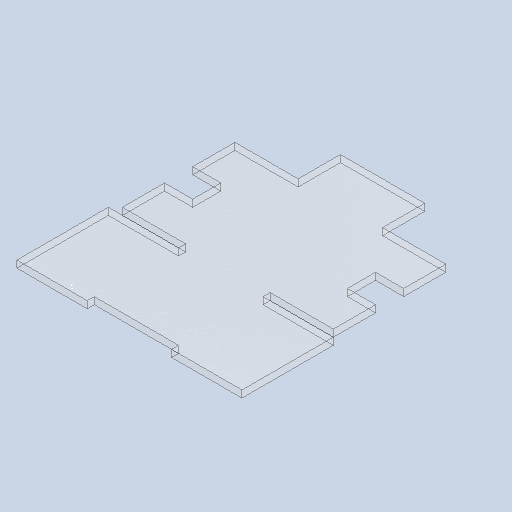
# Autodesk Inventor part: HOOD_1
Saved by Autodesk Inventor 2025.3 (Build 293356030, 356C)
## iProperties
Created: 2026-06-30
Part Number: HOOD_1
Material: Acrylic
Document SubType Name: Modeling
Designer: user
Density: 1.188 g/cm^3
Appearance: Transparent - Clear
Author: user
Autodesk Inventor part; units mm, degrees
ref_plane "YZ Plane" through (0, 0, 0) normal (1, 0, 0) x (0, 1, 0)
ref_plane "XZ Plane" through (0, 0, 0) normal (0, 1, 0) x (-1, 0, 0)
ref_plane "XY Plane" through (0, 0, 0) normal (0, 0, 1) x (1, 0, 0)
sketch "Sketch1" plane through (0, 0, 0) normal (0, 1, 0) x (-1, 0, 0)
  line L0 (150, -70) -> (150, -180)
  line L1 (150, -180) -> (0, -180)
  line L2 (0, -180) -> (0, -70)
  line L3 (45, -180) -> (105, -180)
  line L4 (0, -70) -> (150, -70)
  line L5 (0, -70) -> (50, -70)
  line L6 (150, -70) -> (110, -70)
  line L7 (150, -120) -> (130, -120)
  line L8 (130, -120) -> (130, -100)
  line L9 (130, -100) -> (150, -100)
  line L10 (150, -100) -> (150, -120)
  line L11 (0, -120) -> (20, -120)
  line L12 (20, -120) -> (20, -100)
  line L13 (20, -100) -> (0, -100)
  line L14 (0, -150) -> (150, -150) construction
  line L15 (45, -150) -> (105, -150)
  line L16 (105, -150) -> (105, -180)
  line L17 (105, -180) -> (45, -180)
  line L18 (45, -180) -> (45, -150)
  line L19 (105, -180) -> (45, -180)
  line L20 (150, -150) -> (105, -150)
  line L21 (45, -150) -> (0, -150)
  line L22 (130, 0) -> (150, 0)
  line L23 (155, -70) -> (-5, -70)
  line L24 (-5, -70) -> (-5, 0)
  line L25 (-5, 0) -> (155, 0)
  line L26 (155, 0) -> (155, -70)
  line L27 (75, -180) -> (75, 0) construction
  line L28 (-5, -70) -> (45, -70)
  line L29 (45, -70) -> (45, -65)
  line L30 (45, -65) -> (-5, -65)
  line L31 (-5, -65) -> (-5, -70)
  line L32 (150, -70) -> (100, -70)
  line L33 (155, -70) -> (105, -70)
  line L34 (105, -70) -> (105, -65)
  line L35 (105, -65) -> (155, -65)
  line L36 (155, -65) -> (155, -70)
  line L37 (105, 0) -> (45, 0)
  line L38 (45, 0) -> (45, -5)
  line L39 (45, -5) -> (105, -5)
  line L40 (105, -5) -> (105, 0)
  point P0 (0, 0)
  point P1 (130, -70)
  point P2 (150, -100)
  point P3 (45, -180)
  point P4 (-5, -65)
  dimension "d10" = 20
  dimension "d11" = 20
  dimension "d18" = 150
  dimension "d19" = 160
  dimension "d20" = 80
  dimension "d21" = 45
  dimension "d22" = 45
  dimension "d23" = 50
  dimension "d24" = 5
  dimension "d25" = 5
  constraints: 82 end point, 12 parallel, 9 perpendicular, 8 horizontal, 8 point on line, 4 symmetric about line, 3 collinear, 3 midpoint
  measures "d10" distance of L8.end L9.end
  measures "d11" distance of L7.end L8.end
  measures "d18" distance of L14.start L14.end
  measures "d19" distance of L24.end L25.end
  measures "d20" distance between parallel lines of L24 L27
  measures "d21" distance between parallel lines of L2 L18
  measures "d22" distance between parallel lines of L0 L16
  measures "d23" distance of L30.end L29.end
  measures "d24" distance of L29.end L28.end
  measures "d25" distance of L38.end L37.end
extrude "Extrusion1" add sketch "Sketch1" along normal blind 5 contours L0 L9 L8 L7 L20 L15 L21 L2 L11 L12 L13 L4 | L4 L29 L30 L24 L25 L38 L39 L40 L22 L26 L35 L34 | L16 L1 L18 L15
body "Solid1"
